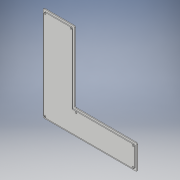
# Autodesk Inventor part: Main Body Lid Backwards
Saved by Autodesk Inventor 2019 (Build 230136000, 136)
## iProperties
Created: 2018-05-20
Part Number: Main Body Lid Backwards
Material: Generic
Document SubType Name: Modeling
Designer: samps
Density: 1 g/cm^3
Appearance: Default
Author: samps
Autodesk Inventor part; units mm, degrees
ref_plane "YZ Plane" through (0, 0, 0) normal (1, 0, 0) x (0, 1, 0)
ref_plane "XZ Plane" through (0, 0, 0) normal (0, 1, 0) x (-1, 0, 0)
ref_plane "XY Plane" through (0, 0, 0) normal (0, 0, 1) x (1, 0, 0)
sketch "Sketch1" plane through (0, 0, 0) normal (0, 0, 1) x (1, 0, 0)
  line L0 (0, 0) -> (3.175, 0)
  line L1 (3.175, 0) -> (53.975, 0)
  line L2 (53.975, 0) -> (57.15, 0)
  line L3 (57.15, 0) -> (57.15, -127)
  line L4 (57.15, -127) -> (111.887, -127)
  line L5 (111.887, -127) -> (169.799, -127)
  line L6 (169.799, -127) -> (169.799, -130.175)
  line L7 (169.799, -130.175) -> (169.799, -168.275)
  line L8 (169.799, -168.275) -> (169.799, -171.45)
  line L9 (169.799, -171.45) -> (57.15, -171.45)
  line L10 (57.15, -171.45) -> (0, -171.45)
  line L11 (0, -171.45) -> (0, 0)
  dimension "d0" = 3.175
  dimension "d1" = 50.8
  dimension "d2" = 3.175
  dimension "d3" = 127
  dimension "d4" = 54.737
  dimension "d5" = 57.912
  dimension "d6" = 3.175
  dimension "d7" = 38.1
  dimension "d8" = 3.175
  constraints: 24 end point, 5 point on line, 4 perpendicular, 2 horizontal, 1 vertical
  measures "d0" distance of L0.start L0.end
  measures "d1" distance of L0.end L1.end
  measures "d2" distance of L1.end L2.end
  measures "d3" distance of L2.end L3.end
  measures "d4" distance of L3.end L4.end
  measures "d5" distance of L4.end L5.end
  measures "d6" distance of L5.end L6.end
  measures "d7" distance of L6.end L7.end
  measures "d8" distance of L7.end L8.end
extrude "Extrusion1" add sketch "Sketch1" along normal blind 1.5875
sketch "Sketch2" plane through (0, 0, 1.5875) normal (0, 0, 1) x (1, 0, 0)
  line L0 (57.15, 0) -> (0, 0) projected
  line L1 (0, 0) -> (0, -171.45) projected
  line L2 (0, -171.45) -> (169.799, -171.45) projected
  line L3 (169.799, -171.45) -> (169.799, -127) projected
  line L4 (169.799, -127) -> (57.15, -127) projected
  line L5 (3.175, -3.175) -> (3.175, -168.275)
  line L6 (3.175, -168.275) -> (166.624, -168.275)
  line L7 (166.624, -168.275) -> (166.624, -130.175)
  line L8 (166.624, -130.175) -> (53.975, -130.175)
  line L9 (53.975, -130.175) -> (53.975, -3.175)
  line L10 (3.175, -3.175) -> (53.975, -3.175)
  constraints: 12 end point, 1 parallel
extrude "Extrusion2" add sketch "Sketch2" along normal blind 1.5875
sketch "Sketch3" plane through (0, 0, 0) normal (0, 0, -1) x (-1, 0, 0)
  line L0 (-169.799, -127) -> (-57.15, -127) projected
  line L1 (-57.15, -127) -> (-57.15, -130.175)
  line L2 (-53.975, -130.175) -> (-166.624, -130.175) projected
  line L3 (-57.15, -130.175) -> (-61.55, -130.175)
  line L4 (-61.55, -130.175) -> (-61.55, -132.325)
  line L5 (-166.624, -168.275) -> (-166.624, -130.175) projected
  line L6 (-166.624, -130.175) -> (-164.474, -130.175)
  line L7 (-164.474, -130.175) -> (-164.474, -132.325)
  line L8 (-166.624, -168.275) -> (-3.175, -168.275) projected
  line L9 (-166.624, -168.275) -> (-164.474, -168.275)
  line L10 (-164.474, -168.275) -> (-164.474, -166.125)
  line L11 (-3.175, -168.275) -> (-3.175, -3.175) projected
  line L12 (-3.175, -168.275) -> (-5.325, -168.275)
  line L13 (-5.325, -168.275) -> (-5.325, -166.125)
  line L14 (-3.175, -3.175) -> (-5.325, -3.175)
  line L15 (-3.175, -3.175) -> (-53.975, -3.175) projected
  line L16 (-5.325, -3.175) -> (-5.325, -5.325)
  line L17 (-53.975, -3.175) -> (-51.825, -3.175)
  line L18 (-51.825, -3.175) -> (-51.825, -5.325)
  point P0 (0, 0)
  dimension "d23" = 4.4
  dimension "d24" = 2.15
  dimension "d25" = 270
  dimension "d26" = 2.15
  dimension "d27" = 2.15
  dimension "d28" = 2.15
  dimension "d29" = 2.15
  dimension "d30" = 2.15
  dimension "d31" = 2.15
  dimension "d32" = 2.15
  dimension "d33" = 2.15
  dimension "d34" = 2.15
  constraints: 26 end point, 7 point on line, 5 perpendicular, 2 vertical
  measures "d23" distance of L1.end L3.end
  measures "d24" distance of L3.end L4.end
  measures "d26" distance of L2.end L6.end
  measures "d27" distance of L6.end L7.end
  measures "d28" distance of L5.start L9.end
  measures "d29" distance of L9.end L10.end
  measures "d30" distance of L8.end L12.end
  measures "d31" distance of L11.end L14.end
  measures "d32" distance of L14.end L16.end
  measures "d33" distance of L15.end L17.end
  measures "d34" distance of L17.end L18.end
hole "Hole1" at (51.825, -5.325, 0) at (5.325, -5.325, 0) at (61.55, -132.325, 0) at (5.325, -166.125, 0) at (164.474, -166.125, 0) at (164.474, -132.325, 0) direction (0, 0, 1) diameter 3 depth 3.175
fillet "Fillet1" radius 2 11 edges at (169.799, -127, 0.7937) (166.624, -130.175, 2.3812) (166.624, -168.275, 2.3812) (169.799, -171.45, 0.7937) (57.15, -127, 0.7937) (3.175, -168.275, 2.3812) (0, -171.45, 0.7937) (57.15, 0, 0.7937) (53.975, -3.175, 2.3812) (3.175, -3.175, 2.3812) (0, 0, 0.7937)
body "Solid1"
